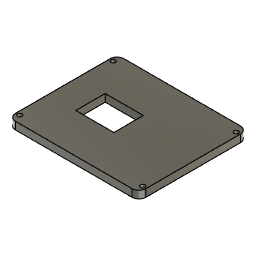
cricket (Autodesk Fusion 360 design; units mm, degrees)
Autodesk Fusion 360 part; units mm, degrees
sketch "pcb" plane through (0, 0, 0) normal (0, 0, 1) x (1, 0, 0)
  line L0 (0, 0) -> (50, 0)
  line L1 (50, 0) -> (50, 40.5)
  line L2 (50, 40.5) -> (0, 40.5)
  line L3 (-3.25, 30.75) -> (0, 30.75)
  line L4 (0, 5) -> (-3.25, 5)
  line L5 (-3.25, 5) -> (-3.25, 30.75)
  line L6 (0, 40.5) -> (0, 30.75)
  line L7 (0, 5) -> (0, 0)
  line L8 (0, 37) -> (50, 37) construction
  line L9 (10, 40.5) -> (10, 0) construction
  circle A0 centre (10, 37) radius 2.625
  line L10 (0, 30.75) -> (0, 5)
  line L11 (-3.25, 5) -> (-3.25, -3.25)
  line L12 (-3.25, -3.25) -> (53.25, -3.25)
  line L13 (53.25, -3.25) -> (53.25, 43.75)
  line L14 (53.25, 43.75) -> (-3.25, 43.75)
  line L15 (-3.25, 43.75) -> (-3.25, 30.75)
  point P0 (10, 37)
  dimension "d1" = 50
  dimension "d2" = 40.5
  dimension "d3" = 3.25
  dimension "d4" = 25.75
  dimension "d5" = 5
  dimension "d6" = 3.5
  dimension "d7" = 10
  dimension "d8" = 5.25
  dimension "d11" = 3.25
  constraint horizontal L0
  constraint vertical L1
  constraint horizontal L2
  constraint vertical L6
  constraint coincident L0.start L7.end
  constraint horizontal L3
  constraint horizontal L4
  constraint vertical L5
  constraint collinear L6 L7
  constraint coincident L6 L8.start
  constraint coincident L1 L8.end
  constraint perpendicular L1 L8
  constraint coincident L2 L9.start
  constraint coincident L0 L9.end
  constraint perpendicular L0 L9
  constraint coincident L9 P0
  constraint coincident L8 P0
  constraint coincident P0 A0.centre
  measures "d1" distance of L0.start L0.end
  measures "d2" distance of L0.start L2.end
  measures "d3" distance of L3.start L3.end
  measures "d4" distance of L3.start L4.end
  measures "d5" distance of L0 L4
  measures "d6" distance of L2 L8
  measures "d7" distance of L6 L9
  measures "d8" diameter of A0
extrude "Extrude2" add sketch "pcb" along normal blind 2 contours L0 L1 L2 L6 L7 L10 | L0 L1 L2 L3 L4 L6 L7 L11 L12 L13 L14 L15 | L3 L4 L5 L10 | A0 makes body 1
extrude "Extrude3" add sketch "pcb" along normal blind 15 from surface at 2 contours L0 L1 L2 L3 L4 L6 L7 L11 L12 L13 L14 L15 bodies 1
extrude "Extrude4" add sketch "pcb" along normal blind 7 from surface at 17 contours L0 L1 L2 L3 L4 L6 L7 L11 L12 L13 L14 L15 | L3 L4 L5 L10 bodies 1
sketch "holes" plane through (0, 0, 2) normal (0, 0, 1) x (-1, 0, 0)
  line L0 (0, -30.75) -> (3.25, -30.75)
  line L1 (3.25, -30.75) -> (3.25, -5)
  line L2 (3.25, -5) -> (0, -5)
  line L3 (0, -5) -> (0, 0)
  line L4 (0, 0) -> (-50, 0)
  line L5 (-50, 0) -> (-50, -40.5)
  line L6 (-50, -40.5) -> (0, -40.5)
  line L7 (0, -40.5) -> (0, -30.75)
  line L8 (-53.25, 3.25) -> (-53.25, -43.75)
  line L9 (-53.25, -43.75) -> (3.25, -43.75)
  line L10 (3.25, -43.75) -> (3.25, 3.25)
  line L11 (3.25, 3.25) -> (-53.25, 3.25)
  line L12 (-50, 0) -> (0, 0)
  line L13 (0, 0) -> (0, -40.5)
  line L14 (0, -40.5) -> (-50, -40.5)
  line L15 (-50, -40.5) -> (-50, 0)
  line L16 (-25, -43.75) -> (-25, 3.25) construction
  line L17 (-53.25, -20.25) -> (3.25, -20.25) construction
  line L18 (0, -40.5) -> (3.25, -40.5) construction
  circle A0 centre (1.625, -40.5) radius 0.975
  circle A1 centre (-51.625, -40.5) radius 0.975
  circle A2 centre (-51.625, 0) radius 0.975
  circle A3 centre (1.625, 0) radius 0.975
  point P0 (1.625, -40.5)
  dimension "d24" = 1.95
  constraint midpoint L9 L16.start
  constraint midpoint L11 L16.end
  constraint midpoint L8 L17.start
  constraint midpoint L10 L17.end
  constraint coincident L6.end L7.start
  constraint coincident L10 L18.end
  constraint perpendicular L10 L18
  constraint midpoint L18 P0
  constraint coincident P0 A0.centre
  constraint symmetric L16 A0 A1
  constraint symmetric L17 A0 A3
  constraint symmetric L17 A1 A2
  measures "d24" diameter of A0
extrude "Extrude6" cut sketch "holes" against normal blind 6 from surface at 22 contours A0 | A1 | A2 | A3 bodies 1
fillet "Fillet1" radius 3 4 edges at (53.25, 43.75, 12) (-3.25, 43.75, 12) (-3.25, -3.25, 12) (53.25, -3.25, 12) on bodies 1
extrude "Extrude8" add sketch "pcb" along normal blind 3.25 from surface at 24 separate body contours L0 L1 L2 L6 L7 L10 | L0 L1 L2 L3 L4 L6 L7 L11 L12 L13 L14 L15 | L3 L4 L5 L10 | A0 makes body 2
move_body "Move1" bodies 2 to x (1, 0, 0) y (0, 1, 0) z (0, 0, 1) at (0, 0, 1)
fillet "Fillet2" radius 3 4 edges at (-3.25, -3.25, 26.625) (-3.25, 43.75, 26.625) (53.25, -3.25, 26.625) (53.25, 43.75, 26.625) on bodies 2
extrude "Extrude9" cut sketch "holes" against normal blind 4 from surface at 26.25 contours A0 | A1 | A2 | A3 bodies 2
sketch "dht" plane through (0, 0, 28.25) normal (0, 0, 1) x (-1, 0, 0)
  circle A0 centre (-51.625, 0) radius 0.975
  circle A1 centre (-51.625, -40.5) radius 0.975
  circle A2 centre (1.625, 0) radius 0.975
  circle A3 centre (1.625, -40.5) radius 0.975
  arc A4 (-53.25, -40.75) -> (-50.25, -43.75) centre (-50.25, -40.75) ccw
  line L0 (-50.25, -43.75) -> (0.25, -43.75)
  arc A5 (0.25, -43.75) -> (3.25, -40.75) centre (0.25, -40.75) ccw
  line L1 (3.25, -40.75) -> (3.25, 0.25)
  arc A6 (3.25, 0.25) -> (0.25, 3.25) centre (0.25, 0.25) ccw
  line L2 (0.25, 3.25) -> (-50.25, 3.25)
  arc A7 (-50.25, 3.25) -> (-53.25, 0.25) centre (-50.25, 0.25) ccw
  line L3 (-53.25, 0.25) -> (-53.25, -40.75)
  line L4 (-25.25, -13.875) -> (-8.75, -13.875)
  line L5 (-8.75, -13.875) -> (-8.75, -26.625)
  line L6 (-8.75, -26.625) -> (-25.25, -26.625)
  line L7 (-25.25, -26.625) -> (-25.25, -13.875)
  line L8 (-53.25, -20.25) -> (3.25, -20.25) construction
  line L9 (-25.25, -20.25) -> (-8.75, -20.25)
  point P0 (-8.75, -20.25)
  dimension "d41" = 16.5
  dimension "d42" = 12.75
  dimension "d43" = 12
  constraint horizontal L4
  constraint vertical L5
  constraint horizontal L6
  constraint vertical L7
  constraint midpoint L3 L8.start
  constraint midpoint L1 L8.end
  constraint midpoint L7 L9.start
  constraint midpoint L5 P0
  constraint coincident P0 L9.end
  constraint coincident L8 P0
  measures "d41" distance of L4.start L4.end
  measures "d42" distance of L4.start L6.end
  measures "d43" distance of L1 L5
extrude "Extrude10" cut sketch "dht" against normal blind 4 contours L4 L5 L7 L9 | L5 L6 L7 L9 bodies 2
hidden bodies 1
named bodies: "main", "lid"
